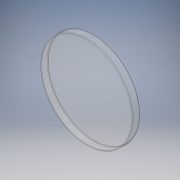
# Autodesk Inventor part: cap_v2
Saved by Autodesk Inventor 2019 (Build 230136000, 136)
## iProperties
Created: 2019-05-09
Part Number: cap_v2
Material: Generic
Document SubType Name: Modeling
Designer: assman
Density: 1 g/cm^3
Appearance: Polycarbonate - Clear
Author: assman
## iProperties of the stored document cap_v2_3DPrint.ipt
Created: 2019-05-09
Part Number: cap_v2_3DPrint
Material: Generic
Document SubType Name: Modeling
Designer: assman
Density: 1 g/cm^3
Appearance: Default
Author: assman
Autodesk Inventor part; units mm, degrees
ref_plane "YZ Plane" through (0, 0, 0) normal (1, 0, 0) x (0, 1, 0)
ref_plane "XZ Plane" through (0, 0, 0) normal (0, 1, 0) x (-1, 0, 0)
ref_plane "XY Plane" through (0, 0, 0) normal (0, 0, 1) x (1, 0, 0)
sketch "Sketch1" plane through (0, 0, 0) normal (0, 0, 1) x (1, 0, 0)
  circle A0 centre (0, 0) radius 100 construction
  circle A1 centre (0, 0) radius 100.1
  circle A2 centre (0, 0) radius 102.1
  point P0 (0, 0)
  dimension "d0" = 0.1
  dimension "d1" = 2
  constraints: 2 centre point
  measures "d0" radial gap between concentric circles of A0 A1
  measures "d1" radial gap between concentric circles of A1 A2
extrude "Extrusion1" add sketch "Sketch1" against normal blind 15
sketch "Sketch2" plane through (0, 0, 0) normal (0, 0, 1) x (1, 0, 0)
  circle A0 centre (0, 0) radius 102.1 projected
  point P0 (0, 0)
extrude "Extrusion2" add sketch "Sketch2" along normal blind 2
fillet "Fillet1" radius 1 1 edges at (-102.1, 0, -15)
fillet "Fillet1" radius 2 1 edges at (-102.1, 0, 2)
body "Solid1"
